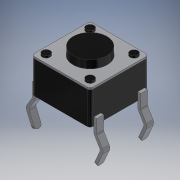
# Autodesk Inventor part: TACT-SWITCH-THT-06X06MM
Saved by Autodesk Inventor 2018.3 (Build 223284000, 284)
## iProperties
Created: 2020-10-19
Part Number: TACT-SWITCH-THT-06X06MM
Material: Genérico
Document SubType Name: Modeling
Designer: laguerre
Density: 8.47 g/cm^3
Appearance: Suave - Negro
Author: laguerre
Autodesk Inventor part; units mm, degrees
ref_plane "YZ Plane" through (0, 0, 0) normal (1, 0, 0) x (0, 1, 0)
ref_plane "XZ Plane" through (0, 0, 0) normal (0, 1, 0) x (-1, 0, 0)
ref_plane "XY Plane" through (0, 0, 0) normal (0, 0, 1) x (1, 0, 0)
sketch "Boceto39" plane through (0, 0, 0) normal (0, 0, 1) x (1, 0, 0)
  line L0 (-2.7, 3) -> (2.7, 3)
  line L1 (3, 2.7) -> (3, -2.7)
  line L2 (2.7, -3) -> (-2.7, -3)
  line L3 (-3, -2.7) -> (-3, 2.7)
  arc A0 (3, 2.7) -> (2.7, 3) centre (2.7, 2.7) ccw
  arc A1 (-2.7, 3) -> (-3, 2.7) centre (-2.7, 2.7) ccw
  arc A2 (-3, -2.7) -> (-2.7, -3) centre (-2.7, -2.7) ccw
  arc A3 (2.7, -3) -> (3, -2.7) centre (2.7, -2.7) ccw
  point P0 (0, 0)
  point P1 (-3, 3)
  point P2 (3, -3)
  point P3 (3, 3)
  point P4 (-3, -3)
  point P5 (0, 3)
  point P6 (3, 0)
  dimension "d373" = 6
  dimension "d376" = 0.3
  constraints: 8 end point, 8 point on circle, 8 point on line, 8 tangent, 4 centre point, 3 equal radius, 2 midpoint, 2 parallel, 2 perpendicular, 1 horizontal, 1 horizontal alignment, 1 vertical alignment
  measures "d373" distance of point (-3, 3) point (3, 3)
  measures "d376" radius of A0
extrude "Extrusión13" add sketch "Boceto39" along normal blind 3.3
sketch "Boceto40" plane through (0, 0, 3.3) normal (0, 0, 1) x (1, 0, 0)
  line L0 (2.7, 3) -> (-2.7, 3) projected
  arc A0 (-2.7, 3) -> (-3, 2.7) centre (-2.7, 2.7) ccw projected
  line L1 (-3, 2.7) -> (-3, -2.7) projected
  arc A1 (-3, -2.7) -> (-2.7, -3) centre (-2.7, -2.7) ccw projected
  line L2 (-2.7, -3) -> (2.7, -3) projected
  arc A2 (2.7, -3) -> (3, -2.7) centre (2.7, -2.7) ccw projected
  line L3 (3, -2.7) -> (3, 2.7) projected
  arc A3 (3, 2.7) -> (2.7, 3) centre (2.7, 2.7) ccw projected
  point P0 (0, 0)
extrude "Extrusión14" add sketch "Boceto40" along normal blind 0.2 separate body
sketch "Boceto43" plane through (0, 0, 0) normal (1, 0, 0) x (0, 1, 0)
  line L0 (0, 0) -> (0, -3.6276) construction
  line L1 (3, 0) -> (3, 3.3) construction
  line L2 (3, 0.8) -> (3, -0.5631)
  line L3 (3.0698, -0.8178) -> (3.6129, -1.7351)
  line L4 (3.6248, -1.9153) -> (3, -3.3825)
  line L5 (3, -3.3825) -> (3.276, -3.5)
  line L6 (3.276, -3.5) -> (3.9008, -2.0329)
  line L7 (3.871, -1.5822) -> (3.3279, -0.665)
  line L8 (3.3, -0.5631) -> (3.3, 0.8)
  line L9 (3.3, 0.8) -> (3, 0.8)
  line L10 (2.7, 3.5) -> (-2.7, 3.5) projected
  line L11 (2.7, 0) -> (-2.7, 0) projected
  arc A0 (3.6248, -1.9153) -> (3.6129, -1.7351) centre (3.4408, -1.837) ccw
  arc A1 (3.3, -0.5631) -> (3.3279, -0.665) centre (3.5, -0.5631) ccw
  arc A2 (3.9008, -2.0329) -> (3.871, -1.5822) centre (3.4408, -1.837) ccw
  arc A3 (3, -0.5631) -> (3.0698, -0.8178) centre (3.5, -0.5631) ccw
  point P0 (3, -0.7)
  point P1 (4, -1.8)
  dimension "d399" = 2.7
  dimension "d400" = 0.3
  dimension "d401" = 0.3
  dimension "d402" = 0.3
  dimension "d403" = 0.7
  dimension "d404" = 4
  dimension "d405" = 3
  dimension "d406" = 1.8
  dimension "d407" = 3.5
  dimension "d408" = 0.2
  dimension "d409" = 0.5
  constraints: 18 end point, 8 point on circle, 8 tangent, 5 point on line, 4 centre point, 3 perpendicular, 2 equal radius, 2 parallel, 2 vertical
  measures "d399" distance between parallel lines of L9 L10
  measures "d400" distance between parallel lines of L8 L2
  measures "d401" distance between parallel lines of L7 L3
  measures "d402" distance between parallel lines of L6 L4
  measures "d403" distance from line of point (3, -0.7) L11
  measures "d404" distance from line of point (4, -1.8) L0
  measures "d405" distance from line of L0 L4.end
  measures "d406" distance from line of point (4, -1.8) L11
  measures "d407" distance from line of L5.end L11
  measures "d408" radius of A0
  measures "d409" radius of A2
extrude "Extrusión15" add sketch "Boceto43" along normal mid plane 5.2 separate body
sketch "Boceto45" plane through (0, 0, 0) normal (1, 0, 0) x (0, 1, 0)
  line L0 (3, 0.8) -> (3, -0.5631) projected
  line L1 (3, 0.8) -> (3.3, 0.8) projected
  line L2 (3, 0.8) -> (4.0467, 0.8)
  line L3 (4.0467, 0.8) -> (4.0467, -3.761)
  line L4 (4.0467, -3.761) -> (3, -3.761)
  line L5 (3, -3.761) -> (3, 0.8)
  point P0 (0, 0)
  constraints: 8 end point, 2 parallel, 1 horizontal, 1 perpendicular
extrude "Extrusión17" cut sketch "Boceto45" along normal mid plane 3.8 bodies 3
fillet "Empalme44" radius 0.3 4 edges at (2.6, 3.138, -3.4412) (1.9, 3.138, -3.4412) (-1.9, 3.138, -3.4412) (-2.6, 3.138, -3.4412)
mirror "Simetría1" about plane through (0, 0, 0) normal (0, 1, 0) of "Extrusión15", "Extrusión17", "Empalme44" bodies 3
sketch "Boceto46" plane through (0, 0, 3.5) normal (0, 0, 1) x (1, 0, 0)
  line L0 (-2.25, -2.25) -> (2.25, -2.25) construction
  line L1 (2.25, -2.25) -> (2.25, 2.25) construction
  line L2 (2.25, 2.25) -> (-2.25, 2.25) construction
  line L3 (-2.25, 2.25) -> (-2.25, -2.25) construction
  circle A0 centre (-2.25, -2.25) radius 0.4
  circle A1 centre (-2.25, 2.25) radius 0.4
  circle A2 centre (2.25, 2.25) radius 0.4
  circle A3 centre (2.25, -2.25) radius 0.4
  point P0 (0, 0)
  point P1 (0, -2.25)
  point P2 (-2.25, 0)
  dimension "d417" = 0.8
  dimension "d418" = 4.5
  constraints: 8 end point, 4 centre point, 4 coincident, 3 equal radius, 2 midpoint, 2 parallel, 2 perpendicular, 1 horizontal, 1 horizontal alignment, 1 vertical alignment
  measures "d417" diameter of A0
  measures "d418" distance of L1.end L2.end
extrude "Extrusión18" add sketch "Boceto46" along normal blind 0.2 bodies 2
sketch "Boceto48" plane through (0, 0, 0) normal (0, 1, 0) x (-1, 0, 0)
  line L0 (0, 0) -> (0, 17.1627)
  line L1 (-2.7, 3.5) -> (2.7, 3.5) construction
  line L2 (0, 3.5) -> (-1.75, 3.5)
  line L3 (-1.75, 3.5) -> (-1.7221, 4.3)
  line L4 (-1.7221, 4.3) -> (0, 4.3)
  line L5 (0, 4.3) -> (0, 3.5)
  line L6 (-2.7, 0) -> (2.7, 0) projected
  line L7 (-1.75, 3.5) -> (-1.75, 4.1675) construction
  dimension "d422" = 4.3
  dimension "d423" = 3.5
  dimension "d424" = 2
  constraints: 12 end point, 2 perpendicular, 2 point on line, 2 vertical, 1 midpoint
  measures "d422" distance between parallel lines of L6 L4
  measures "d423" vertical distance of L2.end L0
  measures "d424" angle of L7 L3
revolve "Revolución14" add sketch "Boceto48" angle 360 about axis through (0, 0, 0) along (0, 0, 1) bodies 2
